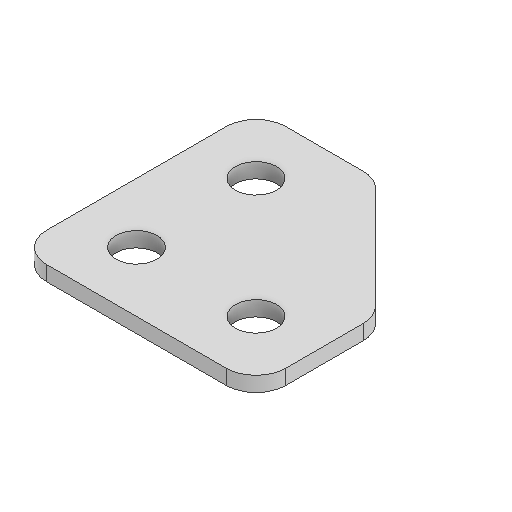
# Autodesk Inventor part: bracket1
Saved by Autodesk Inventor 2023 (Build 270158000, 158)
## iProperties
Created: 2022-12-09
Part Number: bracket1
Material: Generic
Document SubType Name: Modeling
Designer: aaron
Density: 1 g/cm^3
Appearance: Default
Author: aaron
Autodesk Inventor part; units mm, degrees
ref_plane "YZ Plane" through (0, 0, 0) normal (1, 0, 0) x (0, 1, 0)
ref_plane "XZ Plane" through (0, 0, 0) normal (0, 1, 0) x (-1, 0, 0)
ref_plane "XY Plane" through (0, 0, 0) normal (0, 0, 1) x (1, 0, 0)
sketch "Sketch1" plane through (0, 0, 0) normal (0, 1, 0) x (-1, 0, 0)
  line L0 (-12.7, -19.05) -> (12.7, -19.05)
  line L1 (12.7, -19.05) -> (12.7, 19.05)
  line L2 (12.7, 19.05) -> (-12.7, 19.05)
  line L3 (-12.7, 19.05) -> (-12.7, -19.05)
  line L4 (-12.7, -19.05) -> (12.7, 19.05) construction
  line L5 (12.7, -19.05) -> (-12.7, 19.05) construction
  line L6 (12.7, 19.05) -> (0, 19.05)
  line L7 (0, 19.05) -> (0, -19.05)
  line L8 (0, -19.05) -> (12.7, -19.05)
  line L9 (12.7, -19.05) -> (12.7, 19.05)
  line L10 (0, 19.05) -> (-12.7, 6.35)
  line L11 (0, 19.05) -> (17.9605, 19.05) construction
  line L12 (0, -19.05) -> (-12.7, -6.35)
  line L13 (0, -19.05) -> (17.9605, -19.05) construction
  circle A0 centre (6.35, 0) radius 2.1828
  circle A1 centre (-6.35, 0) radius 2.1828
  circle A2 centre (6.35, 12.7) radius 2.1828
  circle A3 centre (6.35, -12.7) radius 2.1828
  point P0 (0, 0)
  point P1 (0, 0)
  point P2 (8.9803, -19.05)
  dimension "d0" = 25.4
  dimension "d1" = 38.1
  dimension "d2" = 135
  dimension "d3" = 135
  dimension "d4" = 4.3656
  dimension "d5" = 4.3656
  dimension "d6" = 4.3656
  dimension "d7" = 4.3656
  dimension "d10" = 12.7
  dimension "d11" = 6.35
  dimension "d12" = 19.05
  dimension "d13" = 19.05
  constraints: 28 end point, 5 midpoint, 4 centre point, 4 horizontal, 4 parallel, 2 equal length, 2 perpendicular, 2 point on line
  measures "d0" distance of L2.end L1.end
  measures "d1" distance of L1.end L0.end
  measures "d2" angle of L10 L11
  measures "d3" angle of L13 L12
  measures "d4" diameter of A0
  measures "d5" diameter of A1
  measures "d6" diameter of A2
  measures "d7" diameter of A3
  measures "d10" distance of A1.centre A0.centre
  measures "d11" distance of A1.centre point (0, 0)
  measures "d12" distance from line of L11 A1.centre
  measures "d13" vertical distance of point (8.98, -19.05) A0.centre
extrude "Extrusion1" add sketch "Sketch1" along normal blind 1.5875 contours L7 L2 L1 L0 | L12 L3 L10 L7
sketch "Sketch2" plane through (0, 1.5875, 0) normal (0, 1, 0) x (1, 0, 0)
  line L0 (12.7, -6.35) -> (12.7, 6.35) projected
  line L1 (12.7, -6.35) -> (-18.9593, -6.35)
  line L2 (-18.9593, -6.35) -> (-18.9593, -20.186)
  line L3 (-18.9593, -20.186) -> (12.7, -20.186)
  line L4 (12.7, -20.186) -> (12.7, -6.35)
  point P0 (0, 0)
  constraints: 8 end point, 2 parallel, 1 horizontal, 1 perpendicular
extrude "Extrusion2" cut sketch "Sketch2" against normal blind 25.4
fillet "Fillet1" radius 3.175 5 edges at (12.7, 0.7937, 6.35) (-12.7, 0.7937, 6.35) (12.7, 0.7937, -6.35) (0, 0.7937, -19.05) (-12.7, 0.7937, -19.05)
body "Solid1"
